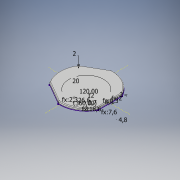
# Autodesk Inventor part: Stewart-Platform-Base-KST-DS215MG
Saved by Autodesk Inventor 2018.2 (Build 222227000, 227)
## iProperties
Created: 2018-02-17
Part Number: Stewart-Platform-Base-KST-DS215MG
Material: Generisch
Document SubType Name: Modeling
Designer: JochenAlt
Density: 1 g/cm^3
Appearance: Vorgabe
Author: JochenAlt
Autodesk Inventor part; units mm, degrees
ref_plane "YZ Plane" through (0, 0, 0) normal (1, 0, 0) x (0, 1, 0)
ref_plane "XZ Plane" through (0, 0, 0) normal (0, 1, 0) x (-1, 0, 0)
sketch "Skizze1" plane through (0, 0, 0) normal (0, 0, 1) x (1, 0, 0)
  line L0 (0, 63.9513) -> (0, -63.9513) construction
  line L1 (-58.3312, 0) -> (67.7052, 0) construction
  line L2 (49.7, 0) -> (47.7, 0) construction
  line L3 (7.0148, -0.15) -> (33.6148, -0.15) construction
  line L4 (33.6148, -0.15) -> (33.6148, -12.15) construction
  line L5 (33.6148, -12.15) -> (7.0148, -12.15) construction
  line L6 (7.0148, -12.15) -> (7.0148, -0.15) construction
  line L7 (7.0148, 0.15) -> (33.6148, 0.15) construction
  line L8 (33.6148, 0.15) -> (33.6148, 12.15) construction
  line L9 (33.6148, 12.15) -> (7.0148, 12.15) construction
  line L10 (7.0148, 12.15) -> (7.0148, 0.15) construction
  line L11 (15.3148, -12.45) -> (15.3148, -17.45)
  line L12 (17.6148, -19.75) -> (31.6148, -19.75)
  line L13 (33.9148, -17.45) -> (33.9148, -12.45)
  line L14 (33.9148, 12.45) -> (33.9148, 17.45)
  line L15 (31.6148, 19.75) -> (17.6148, 19.75)
  line L16 (15.3148, 17.45) -> (15.3148, -4.7068)
  circle A0 centre (18.1148, -16.95) radius 1.35
  circle A1 centre (31.1148, -16.95) radius 1.35
  circle A2 centre (18.1148, 16.95) radius 1.35
  circle A3 centre (31.1148, 16.95) radius 1.35
  line L17 (18.1148, -16.95) -> (31.1148, -16.95) construction
  line L18 (24.6148, -19.75) -> (24.6148, -12.15) construction
  arc A4 (15.3148, -17.45) -> (17.6148, -19.75) centre (17.6148, -17.45) ccw
  arc A5 (31.6148, -19.75) -> (33.9148, -17.45) centre (31.6148, -17.45) ccw
  arc A6 (17.6148, 19.75) -> (15.3148, 17.45) centre (17.6148, 17.45) ccw
  arc A7 (33.9148, 17.45) -> (31.6148, 19.75) centre (31.6148, 17.45) ccw
  line L19 (33.2412, 19.0763) -> (34.9758, 20.0718) construction
  line L20 (33.9148, -12.45) -> (33.9148, 12.45)
  line L21 (15.3148, -12.45) -> (15.3148, -4.7068)
  line L22 (8.2966, 25.1299) -> (1.2966, 37.2542)
  arc A8 (7.4547, 21.988) -> (8.2966, 25.1299) centre (6.3047, 23.9799) ccw
  circle A9 centre (5.6217, 24.1629) radius 1.35
  line L23 (3.1246, 19.488) -> (7.4547, 21.988)
  arc A10 (1.2966, 37.2542) -> (-1.8453, 38.0961) centre (-0.6953, 36.1042) ccw
  line L24 (-1.8453, 38.0961) -> (-6.1754, 35.5961)
  line L25 (3.1246, 19.488) -> (-3.5812, 15.6164)
  line L26 (-32.9114, 17.5042) -> (-25.9114, 5.3799)
  circle A11 centre (-30.2365, 18.4712) radius 1.35
  circle A12 centre (-23.7365, 7.2129) radius 1.35
  arc A13 (-25.9114, 5.3799) -> (-22.7695, 4.538) centre (-23.9195, 6.5299) ccw
  line L27 (-22.7695, 4.538) -> (-3.5812, 15.6164)
  line L28 (-27.7394, 23.1461) -> (-32.0695, 20.6461)
  arc A14 (-32.0695, 20.6461) -> (-32.9114, 17.5042) centre (-30.9195, 18.6542) ccw
  line L29 (-6.1754, 35.5961) -> (-27.7394, 23.1461)
  circle A15 centre (-0.8783, 35.4212) radius 1.35
  line L30 (-25.9114, -5.3799) -> (-32.9114, -17.5042)
  arc A16 (-22.7695, -4.538) -> (-25.9114, -5.3799) centre (-23.9195, -6.5299) ccw
  circle A17 centre (-23.7365, -7.2129) radius 1.35
  line L31 (-18.4394, -7.038) -> (-22.7695, -4.538)
  arc A18 (-32.9114, -17.5042) -> (-32.0695, -20.6461) centre (-30.9195, -18.6542) ccw
  line L32 (-32.0695, -20.6461) -> (-27.7394, -23.1461)
  line L33 (-18.4394, -7.038) -> (-11.7336, -10.9096)
  line L34 (1.2966, -37.2542) -> (8.2966, -25.1299)
  circle A19 centre (-0.8783, -35.4212) radius 1.35
  circle A20 centre (5.6217, -24.1629) radius 1.35
  arc A21 (8.2966, -25.1299) -> (7.4547, -21.988) centre (6.3047, -23.9799) ccw
  line L35 (7.4547, -21.988) -> (-11.7336, -10.9096)
  line L36 (-6.1754, -35.5961) -> (-1.8453, -38.0961)
  arc A22 (-1.8453, -38.0961) -> (1.2966, -37.2542) centre (-0.6953, -36.1042) ccw
  line L37 (-27.7394, -23.1461) -> (-6.1754, -35.5961)
  circle A23 centre (-30.2365, -18.4712) radius 1.35
  line L38 (0, 0) -> (7.0148, -12.15) construction
  line L39 (0, 0) -> (7.0148, 12.15) construction
  line L40 (35.9148, 17.8512) -> (35.9148, -17.8512)
  line L41 (-33.417, 22.1775) -> (-2.4978, 40.0288)
  line L42 (-33.417, -22.1775) -> (-2.4978, -40.0288)
  arc A24 (-34.1087, 21.5124) -> (-34.1087, -21.5124) centre (0, 0) ccw
  arc A25 (-1.5759, -40.2952) -> (35.6846, -18.7828) centre (0, 0) ccw
  arc A26 (35.6846, 18.7828) -> (-1.5759, 40.2952) centre (0, 0) ccw
  arc A27 (-33.417, 22.1775) -> (-34.1087, 21.5124) centre (-32.417, 20.4455) ccw
  arc A28 (-1.5759, 40.2952) -> (-2.4978, 40.0288) centre (-1.4978, 38.2967) ccw
  arc A29 (35.9148, 17.8512) -> (35.6846, 18.7828) centre (33.9148, 17.8512) ccw
  arc A30 (35.6846, -18.7828) -> (35.9148, -17.8512) centre (33.9148, -17.8512) ccw
  arc A31 (-2.4978, -40.0288) -> (-1.5759, -40.2952) centre (-1.4978, -38.2967) ccw
  arc A32 (-34.1087, -21.5124) -> (-33.417, -22.1775) centre (-32.417, -20.4455) ccw
  circle A33 centre (0, 0) radius 10
  point P0 (15.3148, -19.75)
  point P1 (15.3148, 19.75)
  point P2 (4.7966, 31.192)
  point P3 (9.4466, 23.138)
  point P4 (-24.7614, 3.388)
  point P5 (-33.1412, 19.2495)
  point P6 (-29.4114, -11.442)
  point P7 (-24.7614, -3.388)
  point P8 (9.4466, -23.138)
  point P9 (-0.1, -38.3259)
  point P10 (35.9148, -18.3388)
  point P11 (-33.8393, 21.9337)
  point P12 (-2.0755, 40.2725)
  point P13 (-33.8393, -21.9337)
  point P14 (-2.0755, -40.2725)
  point P15 (35.9148, 18.3388)
  dimension "d164" = 12
  dimension "d165" = 26.6
  dimension "d166" = 18.6
  dimension "d169" = 13
  dimension "d170" = 2.7
  dimension "d171" = 4.8
  dimension "d172" = 2.3
  dimension "d173" = 7.6
  dimension "d177" = 2
  dimension "d190" = 0.3
  dimension "d197" = 360
  dimension "d199" = 120
  dimension "d200" = 2
  dimension "d201" = 0.3
  dimension "d202" = 2
  dimension "d204" = 20
  dimension "d73" = 120
  dimension "d89" = 20
  dimension "d90" = 4
  dimension "d91" = 3.3
  dimension "d146" = 3
  dimension "d147" = 4.2
  constraints: 82 end point, 50 point on circle, 34 centre point, 21 point on line, 20 tangent, 12 equal radius, 8 symmetric about line, 6 parallel, 5 perpendicular, 4 midpoint, 3 line through centre, 2 coincident, 2 collinear, 1 equal length, 1 vertical, 125 other
  measures "d164" distance between parallel lines of L3 L5
  measures "d165" distance between parallel lines of L6 L4
  measures "d166" distance between parallel lines of L13 L11
  measures "d169" distance of L17.end L17.start
  measures "d170" diameter of A0
  measures "d171" distance between parallel lines of L5 L17
  measures "d172" radius of A4
  measures "d173" distance between parallel lines of L5 L12
  measures "d177" distance of L19.start L19.end
  measures "d190" distance between parallel lines of L7 L3
  measures "d199" angle of L39 L38
  measures "d200" distance between parallel lines of L14 L40
  measures "d201" distance between parallel lines of L20 L8
  measures "d202" radius of A27
  measures "d204" diameter of A33
extrude "Extrusion12" add sketch "Skizze1" along normal blind 4 contours L21 L16 A6 L15 A7 L14 L20 L13 A5 L12 A4 L11 | A0 | A1 | A2 | A3 | A8 L23 L25 L27 A13 L26 A14 L28 L29 L24 A10 L22 | A9 | A11 | A12 | A15 | A16 L31 L33 L35 A21 L34 A22 L36 L37 L32 A18 L30 | A17 | A19 | A23 | L40 A30 A25 A31 L42 A32 A24 A27 L41 A28 A26 A29 | A33
extrude "Extrusion5" [suppressed]
extrude "Extrusion4" add sketch "Skizze1" along normal blind 2 contours L21 L16 A6 L15 A7 L14 L20 L13 A5 L12 A4 L11 | A8 L23 L25 L27 A13 L26 A14 L28 L29 L24 A10 L22 | A16 L31 L33 L35 A21 L34 A22 L36 L37 L32 A18 L30
fillet "Rundung3" radius 1 24 edges at (-33.8033, -21.887, 4) (-17.9574, -31.1031, 4) (-2.0531, -40.2181, 4) (20.163, -34.9233, 4) (35.8564, -18.331, 4) (35.9148, 0, 4) (35.8564, 18.331, 4) (20.163, 34.9233, 4) (-2.0531, 40.2181, 4) (-17.9574, 31.1031, 4) (-33.8033, 21.887, 4) (-40.326, 0, 4) (-33.8033, -21.887, 0) (-17.9574, -31.1031, 0) (-2.0531, -40.2181, 0) (20.163, -34.9233, 0) (35.8564, -18.331, 0) (35.9148, 0, 0) (35.8564, 18.331, 0) (20.163, 34.9233, 0) (-2.0531, 40.2181, 0) (-17.9574, 31.1031, 0) (-33.8033, 21.887, 0) (-40.326, 0, 0)
sketch "Skizze7" plane through (34.1, 8.75, -40.8) normal (1, 0, 0) x (0, 0, -1)
  circle A0 centre (3.8, -3.7) radius 1.7
  circle A1 centre (3.8, -13.8) radius 1.7
  line L0 (0, -17.5) -> (0, 0) construction
  line L1 (0, -8.75) -> (7.1, -8.75) construction
  line L2 (7.1, 0) -> (7.1, -17.5) construction
  point P0 (-40.8, -8.75)
  dimension "d76" = 3.4
  dimension "d77" = 10.1
  dimension "d88" = 3.3
  constraints: 2 centre point, 2 end point, 2 midpoint, 1 equal radius, 1 symmetric about line
  measures "d76" diameter of A1
  measures "d77" distance of A0.centre A1.centre
  measures "d88" distance from line of A0.centre L2
sketch "Skizze8" plane through (0, 0, 4) normal (0, 0, 1) x (1, 0, 0)
  circle A0 centre (6.3269, -40.1414) radius 1.25 construction
  circle A1 centre (-37.9269, -14.5914) radius 1.25 construction
  circle A2 centre (0.0769, -50.9667) radius 1.25 construction
  circle A3 centre (-44.1769, -25.4167) radius 1.25 construction
  circle A4 centre (-37.9269, 14.5914) radius 1.25 construction
  circle A5 centre (6.3269, 40.1414) radius 1.25 construction
  circle A6 centre (-44.1769, 25.4167) radius 1.25 construction
  circle A7 centre (0.0769, 50.9667) radius 1.25 construction
  circle A8 centre (44.1, -25.55) radius 1.25 construction
  circle A9 centre (31.6, -25.55) radius 1.25 construction
  circle A10 centre (44.1, 25.55) radius 1.25 construction
  circle A11 centre (31.6, 25.55) radius 1.25 construction
  line L0 (-13.1223, -40.2285) -> (-28.2777, -31.4785) construction
  line L1 (-30.7026, -30.0785) -> (-38.237, -25.7285) construction
  line L2 (-38.237, -25.7285) -> (-36.687, -23.0438) construction
  line L3 (-36.687, -23.0438) -> (-1.613, -43.2938) construction
  line L4 (-1.613, -43.2938) -> (-3.163, -45.9785) construction
  line L5 (-28.2777, 31.4785) -> (-13.1223, 40.2285) construction
  line L6 (-10.6974, 41.6285) -> (-3.163, 45.9785) construction
  line L7 (-3.163, 45.9785) -> (-1.613, 43.2938) construction
  line L8 (-1.613, 43.2938) -> (-36.687, 23.0438) construction
  line L9 (-36.687, 23.0438) -> (-38.237, 25.7285) construction
  line L10 (41.4, 20.25) -> (41.4, 11.55) construction
  line L11 (38.3, -20.25) -> (38.3, 20.25) construction
  line L12 (38.3, 20.25) -> (41.4, 20.25) construction
  line L13 (41.4, -11.55) -> (41.4, -20.25) construction
  line L14 (41.4, -20.25) -> (38.3, -20.25) construction
  line L15 (41.4, -11.55) -> (44.416, -11.55) projected
  line L16 (41.4, 8.75) -> (44.416, 8.75) projected
  line L17 (44.416, 11.55) -> (41.4, 11.55) projected
  line L18 (42.216, 8.75) -> (44.416, 8.75)
  line L19 (44.416, 8.75) -> (44.416, 11.55)
  line L20 (44.416, 11.55) -> (42.216, 11.55)
  line L21 (42.216, 11.55) -> (42.216, 8.75)
  line L22 (-29.7857, -34.0904) -> (-28.2777, -31.4785) projected
  line L23 (-28.6857, -32.1851) -> (-13.5303, -40.9351) construction
  line L24 (-28.6857, 32.1851) -> (-13.5303, 40.9351) construction
  line L25 (-13.1223, 40.2285) -> (-14.6303, 42.8404) construction
  line L26 (-29.7857, 34.0904) -> (-28.2777, 31.4785) projected
  line L27 (-28.6857, 32.1851) -> (-29.7857, 34.0904)
  line L28 (-29.7857, 34.0904) -> (-32.2106, 32.6904)
  line L29 (-32.2106, 32.6904) -> (-31.1106, 30.7851)
  line L30 (-31.1106, 30.7851) -> (-28.6857, 32.1851)
  line L31 (-13.5303, 40.9351) -> (-14.6303, 42.8404)
  line L32 (-14.6303, 42.8404) -> (-12.2054, 44.2404)
  line L33 (-12.2054, 44.2404) -> (-11.1054, 42.3351)
  line L34 (-11.1054, 42.3351) -> (-13.5303, 40.9351)
  line L35 (-13.5303, -40.9351) -> (-14.6303, -42.8404)
  line L36 (-14.6303, -42.8404) -> (-12.2054, -44.2404)
  line L37 (-12.2054, -44.2404) -> (-11.1054, -42.3351)
  line L38 (-11.1054, -42.3351) -> (-13.5303, -40.9351)
  line L39 (-28.6857, -32.1851) -> (-29.7857, -34.0904)
  line L40 (-29.7857, -34.0904) -> (-32.2106, -32.6904)
  line L41 (-32.2106, -32.6904) -> (-31.1106, -30.7851)
  line L42 (-31.1106, -30.7851) -> (-28.6857, -32.1851)
  line L43 (-13.1223, 40.2285) -> (-14.6303, 42.8404) projected
  line L44 (-14.6303, 42.8404) -> (-12.2054, 44.2404) projected
  line L45 (-12.2054, 44.2404) -> (-10.6974, 41.6285) projected
  line L46 (-38.237, 25.7285) -> (-30.7026, 30.0785) projected
  line L47 (-30.7026, 30.0785) -> (-32.2106, 32.6904) projected
  line L48 (-32.2106, 32.6904) -> (-29.7857, 34.0904) projected
  line L49 (-29.7857, 34.0904) -> (-28.2777, 31.4785) projected
  line L50 (41.4, 8.75) -> (41.4, -8.75) projected
  line L51 (41.4, -8.75) -> (44.416, -8.75) projected
  line L52 (44.416, -8.75) -> (44.416, -11.55) projected
  line L53 (44.416, -11.55) -> (41.4, -11.55) projected
  line L54 (41.4, 11.55) -> (44.416, 11.55) projected
  line L55 (44.416, 11.55) -> (44.416, 8.75) projected
  line L56 (44.416, 8.75) -> (41.4, 8.75) projected
  line L57 (-3.163, -45.9785) -> (-10.6974, -41.6285) projected
  line L58 (-10.6974, -41.6285) -> (-12.2054, -44.2404) projected
  line L59 (-12.2054, -44.2404) -> (-14.6303, -42.8404) projected
  line L60 (-14.6303, -42.8404) -> (-13.1223, -40.2285) projected
  line L61 (-28.2777, -31.4785) -> (-29.7857, -34.0904) projected
  line L62 (-29.7857, -34.0904) -> (-32.2106, -32.6904) projected
  line L63 (-32.2106, -32.6904) -> (-30.7026, -30.0785) projected
  arc A12 (44.1, -29.15) -> (47.7, -25.55) centre (44.1, -25.55) ccw construction
  line L64 (47.7, -19.95) -> (41.4, -19.95) construction
  line L65 (41.4, -19.95) -> (41.4, -11.55) construction
  line L66 (41.4, -11.55) -> (44.416, -11.55) construction
  line L67 (44.416, -11.55) -> (44.416, -8.75) construction
  line L68 (44.416, -8.75) -> (41.4, -8.75) construction
  line L69 (41.4, -8.75) -> (41.4, 8.75) construction
  line L70 (41.4, 8.75) -> (44.416, 8.75) construction
  line L71 (44.416, 8.75) -> (44.416, 11.55) construction
  line L72 (44.416, 11.55) -> (41.4, 11.55) construction
  line L73 (41.4, 11.55) -> (41.4, 19.95) construction
  line L74 (41.4, 19.95) -> (47.7, 19.95) construction
  arc A13 (47.7, 25.55) -> (44.1, 29.15) centre (44.1, 25.55) ccw construction
  circle A14 centre (44.1, -25.55) radius 1.25 construction
  circle A15 centre (31.6, -25.55) radius 1.25 construction
  circle A16 centre (44.1, 25.55) radius 1.25 construction
  circle A17 centre (31.6, 25.55) radius 1.25 construction
  line L75 (41.4, 20.25) -> (41.4, 19.95) construction
  line L76 (38.3, 20.25) -> (41.4, 20.25) construction
  line L77 (38.3, -20.25) -> (38.3, 20.25) construction
  line L78 (41.4, -20.25) -> (38.3, -20.25) construction
  line L79 (41.4, -19.95) -> (41.4, -20.25) construction
  line L80 (47.7, -19.95) -> (41.4, -19.95) construction
  line L81 (47.7, -25.55) -> (47.7, -19.95) construction
  arc A18 (44.1, -29.15) -> (47.7, -25.55) centre (44.1, -25.55) ccw construction
  line L82 (31.6, -29.15) -> (44.1, -29.15) construction
  arc A19 (28, -25.55) -> (31.6, -29.15) centre (31.6, -25.55) ccw construction
  line L83 (28, 25.55) -> (28, -25.55) construction
  arc A20 (31.6, 29.15) -> (28, 25.55) centre (31.6, 25.55) ccw construction
  line L84 (44.1, 29.15) -> (31.6, 29.15) construction
  arc A21 (47.7, 25.55) -> (44.1, 29.15) centre (44.1, 25.55) ccw construction
  line L85 (47.7, 19.95) -> (47.7, 25.55) construction
  line L86 (41.4, 19.95) -> (47.7, 19.95) construction
  line L87 (44.416, -8.75) -> (41.4, -8.75) projected
  line L88 (44.416, -8.75) -> (42.216, -8.75)
  line L89 (42.216, -8.75) -> (42.216, -11.55)
  line L90 (42.216, -11.55) -> (44.416, -11.55)
  line L91 (44.416, -11.55) -> (44.416, -8.75)
  line L92 (42.216, 8.75) -> (42.216, -8.75) construction
  line L93 (41.4, -8.75) -> (44.416, -8.75) construction
  line L94 (47.7, 19.95) -> (47.7, 25.55) projected
  line L95 (44.1, 29.15) -> (31.6, 29.15) projected
  arc A22 (31.6, 29.15) -> (28, 25.55) centre (31.6, 25.55) ccw projected
  line L96 (28, 25.55) -> (28, -25.55) projected
  arc A23 (28, -25.55) -> (31.6, -29.15) centre (31.6, -25.55) ccw projected
  line L97 (31.6, -29.15) -> (44.1, -29.15) projected
  line L98 (47.7, -25.55) -> (47.7, -19.95) projected
  arc A24 (-41.0446, 12.7914) -> (-36.1269, 11.4737) centre (-37.9269, 14.5914) ccw projected
  arc A25 (-36.1269, -11.4737) -> (-41.0446, -12.7914) centre (-37.9269, -14.5914) ccw projected
  line L99 (8.1269, -37.0237) -> (-36.1269, -11.4737) projected
  arc A26 (9.4446, -41.9414) -> (8.1269, -37.0237) centre (6.3269, -40.1414) ccw projected
  arc A27 (8.1269, 37.0237) -> (9.4446, 41.9414) centre (6.3269, 40.1414) ccw projected
  line L100 (-36.1269, 11.4737) -> (8.1269, 37.0237) projected
  line L101 (-47.2946, 23.6167) -> (-41.0446, 12.7914) projected
  arc A28 (-45.9769, 28.5344) -> (-47.2946, 23.6167) centre (-44.1769, 25.4167) ccw projected
  line L102 (-41.1272, 31.3344) -> (-45.9769, 28.5344) projected
  line L103 (-37.9772, 25.8785) -> (-41.1272, 31.3344) projected
  line L104 (-38.237, 25.7285) -> (-37.9772, 25.8785) projected
  line L105 (-36.687, 23.0438) -> (-38.237, 25.7285) projected
  line L106 (-1.613, 43.2938) -> (-36.687, 23.0438) projected
  line L107 (-3.163, 45.9785) -> (-1.613, 43.2938) projected
  line L108 (-3.4228, 45.8285) -> (-3.163, 45.9785) projected
  line L109 (-6.5728, 51.2844) -> (-3.4228, 45.8285) projected
  line L110 (-1.7231, 54.0844) -> (-6.5728, 51.2844) projected
  arc A29 (3.1946, 52.7667) -> (-1.7231, 54.0844) centre (0.0769, 50.9667) ccw projected
  line L111 (9.4446, 41.9414) -> (3.1946, 52.7667) projected
  line L112 (3.1946, -52.7667) -> (9.4446, -41.9414) projected
  arc A30 (-1.7231, -54.0844) -> (3.1946, -52.7667) centre (0.0769, -50.9667) ccw projected
  line L113 (-6.5728, -51.2844) -> (-1.7231, -54.0844) projected
  line L114 (-3.4228, -45.8285) -> (-6.5728, -51.2844) projected
  line L115 (-3.163, -45.9785) -> (-3.4228, -45.8285) projected
  line L116 (-1.613, -43.2938) -> (-3.163, -45.9785) projected
  line L117 (-36.687, -23.0438) -> (-1.613, -43.2938) projected
  line L118 (-38.237, -25.7285) -> (-36.687, -23.0438) projected
  line L119 (-37.9772, -25.8785) -> (-38.237, -25.7285) projected
  line L120 (-41.1272, -31.3344) -> (-37.9772, -25.8785) projected
  line L121 (-45.9769, -28.5344) -> (-41.1272, -31.3344) projected
  arc A31 (-47.2946, -23.6167) -> (-45.9769, -28.5344) centre (-44.1769, -25.4167) ccw projected
  line L122 (-41.0446, -12.7914) -> (-47.2946, -23.6167) projected
  arc A32 (8.1269, 37.0237) -> (9.4446, 41.9414) centre (6.3269, 40.1414) ccw projected
  arc A33 (9.4446, -41.9414) -> (8.1269, -37.0237) centre (6.3269, -40.1414) ccw projected
  line L123 (8.1269, -37.0237) -> (-36.1269, -11.4737) projected
  arc A34 (-36.1269, -11.4737) -> (-41.0446, -12.7914) centre (-37.9269, -14.5914) ccw projected
  arc A35 (-41.0446, 12.7914) -> (-36.1269, 11.4737) centre (-37.9269, 14.5914) ccw projected
  line L124 (-36.1269, 11.4737) -> (8.1269, 37.0237) projected
  line L125 (-41.1272, -31.3344) -> (-37.9772, -25.8785) projected
  line L126 (-37.9772, -25.8785) -> (-30.7026, -30.0785) projected
  line L127 (-30.7026, -30.0785) -> (-32.2106, -32.6904) projected
  line L128 (-32.2106, -32.6904) -> (-29.7857, -34.0904) projected
  line L129 (-29.7857, -34.0904) -> (-28.2777, -31.4785) projected
  line L130 (-28.2777, -31.4785) -> (-13.1223, -40.2285) projected
  line L131 (-13.1223, -40.2285) -> (-14.6303, -42.8404) projected
  line L132 (-14.6303, -42.8404) -> (-12.2054, -44.2404) projected
  line L133 (-12.2054, -44.2404) -> (-10.6974, -41.6285) projected
  line L134 (-10.6974, -41.6285) -> (-3.4228, -45.8285) projected
  line L135 (-3.4228, -45.8285) -> (-6.5728, -51.2844) projected
  line L136 (-6.5728, -51.2844) -> (-1.7231, -54.0844) projected
  arc A36 (-1.7231, -54.0844) -> (3.1946, -52.7667) centre (0.0769, -50.9667) ccw projected
  line L137 (3.1946, -52.7667) -> (9.4446, -41.9414) projected
  line L138 (9.4446, 41.9414) -> (3.1946, 52.7667) projected
  arc A37 (3.1946, 52.7667) -> (-1.7231, 54.0844) centre (0.0769, 50.9667) ccw projected
  line L139 (-1.7231, 54.0844) -> (-6.5728, 51.2844) projected
  line L140 (-6.5728, 51.2844) -> (-3.4228, 45.8285) projected
  line L141 (-3.4228, 45.8285) -> (-10.6974, 41.6285) projected
  line L142 (-10.6974, 41.6285) -> (-12.2054, 44.2404) projected
  line L143 (-12.2054, 44.2404) -> (-14.6303, 42.8404) projected
  line L144 (-14.6303, 42.8404) -> (-13.1223, 40.2285) projected
  line L145 (-13.1223, 40.2285) -> (-28.2777, 31.4785) projected
  line L146 (-28.2777, 31.4785) -> (-29.7857, 34.0904) projected
  line L147 (-29.7857, 34.0904) -> (-32.2106, 32.6904) projected
  line L148 (-32.2106, 32.6904) -> (-30.7026, 30.0785) projected
  line L149 (-30.7026, 30.0785) -> (-37.9772, 25.8785) projected
  line L150 (-37.9772, 25.8785) -> (-41.1272, 31.3344) projected
  line L151 (-41.1272, 31.3344) -> (-45.9769, 28.5344) projected
  arc A38 (-45.9769, 28.5344) -> (-47.2946, 23.6167) centre (-44.1769, 25.4167) ccw projected
  line L152 (-47.2946, 23.6167) -> (-41.0446, 12.7914) projected
  line L153 (-41.0446, -12.7914) -> (-47.2946, -23.6167) projected
  arc A39 (-47.2946, -23.6167) -> (-45.9769, -28.5344) centre (-44.1769, -25.4167) ccw projected
  line L154 (-45.9769, -28.5344) -> (-41.1272, -31.3344) projected
  point P0 (0, 0)
  dimension "d142" = 0.816
  dimension "d144" = 0.816
  constraints: 54 end point, 13 parallel, 7 perpendicular, 4 point on line, 2 collinear, 1 horizontal
  measures "d142" distance between parallel lines of L5 L24
  measures "d144" distance between parallel lines of L50 L92
equation "\"d44\" = d21"
equation "\"d21\" = 0.3"
